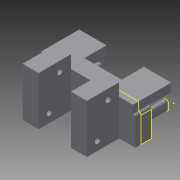
# Autodesk Inventor part: wheelbottomleft
Saved by Autodesk Inventor 2013 SP2 (Build 170200200, 200)
## iProperties
Created: 2015-05-11
Part Number: wheelbottomleft
Document SubType Name: Modeling
Designer: 2016ahoganso
Density: 1 g/cm^3
Material: Generic
Author: 2016ahoganso
Autodesk Inventor part; units mm, degrees
ref_plane "YZ Plane" through (0, 0, 0) normal (1, 0, 0) x (0, 1, 0)
ref_plane "XZ Plane" through (0, 0, 0) normal (0, 1, 0) x (-1, 0, 0)
ref_plane "XY Plane" through (0, 0, 0) normal (0, 0, 1) x (1, 0, 0)
sketch "Sketch1" plane through (0, 0, 0) normal (0, 0, 1) x (1, 0, 0)
  line L0 (2.032, 0) -> (2.032, 0)
  line L1 (4.064, -2.032) -> (4.064, -6.096)
  line L2 (2.032, -8.128) -> (2.032, -8.128)
  line L3 (0, -6.096) -> (0, -2.032)
  arc A0 (2.032, -8.128) -> (4.064, -6.096) centre (2.032, -6.096) ccw
  arc A1 (0, -6.096) -> (2.032, -8.128) centre (2.032, -6.096) ccw
  arc A2 (4.064, -2.032) -> (2.032, 0) centre (2.032, -2.032) ccw
  arc A3 (2.032, 0) -> (0, -2.032) centre (2.032, -2.032) ccw
  line L4 (-8.636, -2.032) -> (-8.636, -6.096)
  line L5 (-12.7, -6.096) -> (-12.7, -2.032)
  arc A4 (-10.668, -8.128) -> (-8.636, -6.096) centre (-10.668, -6.096) ccw
  arc A5 (-12.7, -6.096) -> (-10.668, -8.128) centre (-10.668, -6.096) ccw
  arc A6 (-8.636, -2.032) -> (-10.668, 0) centre (-10.668, -2.032) ccw
  arc A7 (-10.668, 0) -> (-12.7, -2.032) centre (-10.668, -2.032) ccw
  line L6 (8.128, 6.604) -> (-17.018, 6.604)
  line L7 (-17.018, 6.604) -> (-17.018, -15.494)
  line L8 (-17.018, -15.494) -> (8.128, -15.494)
  line L9 (8.128, 6.604) -> (8.128, -15.494)
  line L10 (8.128, -15.494) -> (-17.018, -15.494)
  line L11 (-17.018, -15.494) -> (-17.018, -19.144)
  line L12 (-17.018, -19.144) -> (8.128, -19.144)
  line L13 (8.128, -19.144) -> (8.128, -15.494)
  dimension "d15" = 3.65
  constraints: 28 end point, 16 point on circle, 12 tangent, 8 centre point, 6 parallel, 4 perpendicular, 3 horizontal, 2 equal radius
  measures "d15" distance between parallel lines of L10 L12
surface "Composite1"
surface "Composite2"
surface "Composite3"
surface "Composite4"
surface "Composite5"
surface "Composite6"
surface "Composite7"
surface "Composite8"
surface "Composite9"
surface "Composite10"
extrude "Extrusion2" add sketch "Sketch1" along normal blind 17.526 draft -1 contours L1 A0 A1 L3 A3 A2 | L4 A4 A5 L5 A7 A6
sketch "Sketch2" plane through (0, 0, 17.526) normal (0, 0, 1) x (1, 0, 0)
  line L0 (6.096, 6.858) -> (-15.24, 6.858)
  line L1 (-17.272, 4.826) -> (-17.272, -15.24)
  line L2 (-17.272, -15.24) -> (8.128, -15.24)
  line L3 (8.128, -15.24) -> (8.128, 4.826)
  arc A0 (8.128, 4.826) -> (6.096, 6.858) centre (6.096, 4.826) ccw
  line L4 (0.3059, -6.096) -> (0.3059, -2.032) projected
  line L5 (-17.272, 4.2146) -> (-17.272, 6.858)
  line L6 (-17.272, 6.858) -> (-15.24, 6.858)
  point P0 (0, 0)
  constraints: 12 end point, 3 parallel, 2 point on circle, 2 tangent, 1 centre point, 1 collinear, 1 horizontal, 1 perpendicular, 1 point on line
extrude "Extrusion3" add sketch "Sketch2" along normal blind 6.35
sketch "Sketch3" plane through (0, 0, 23.876) normal (0, 0, 1) x (1, 0, 0)
  line L0 (-15.24, 6.858) -> (6.344, 6.858)
  line L1 (6.344, 6.858) -> (6.344, 13.208)
  line L2 (6.344, 13.208) -> (-15.24, 13.208)
  line L3 (-15.24, 13.208) -> (-15.24, 6.858)
  point P0 (0, 0)
  dimension "d27" = 6.35
  constraints: 8 end point, 2 parallel, 1 horizontal, 1 perpendicular
  measures "d27" distance of L2.end L0.start
extrude "Extrusion4" add sketch "Sketch3" against normal blind 23.876
sketch "Sketch4" plane through (0, 0, 0) normal (0, 0, -1) x (-1, 0, 0)
  arc A0 (-4.064, -6.096) -> (0, -6.096) centre (-2.032, -6.096) ccw projected
  line L0 (0, -6.096) -> (0, -2.032) projected
  arc A1 (0, -2.032) -> (-4.064, -2.032) centre (-2.032, -2.032) ccw projected
  line L1 (-4.064, -2.032) -> (-4.064, -6.096) projected
fillet "Fillet1" radius 1.524 8 edges at (4.064, -4.064, 0) (2.032, -8.128, 0) (0, -4.064, 0) (2.032, 0, 0) (-8.636, -4.064, 0) (-10.668, 0, 0) (-12.7, -4.064, 0) (-10.668, -8.128, 0)
sketch "Sketch5" plane through (0, 0, 23.876) normal (0, 0, 1) x (1, 0, 0)
  arc A0 (-15.24, 6.858) -> (-17.272, 4.826) centre (-15.24, 4.826) ccw projected
  line L0 (-17.272, -15.24) -> (-17.272, 6.858) projected
  line L1 (8.128, -15.24) -> (-17.272, -15.24) projected
  line L2 (8.128, 4.826) -> (8.128, -15.24) projected
  arc A1 (8.128, 4.826) -> (6.096, 6.858) centre (6.096, 4.826) ccw projected
  line L3 (6.096, 6.858) -> (6.344, 6.858) projected
  line L4 (6.344, 6.858) -> (6.344, 13.208) projected
  line L5 (6.344, 13.208) -> (-15.24, 13.208) projected
  line L6 (-15.24, 13.208) -> (-15.24, 6.858) projected
  point P0 (0, 0)
extrude "Extrusion5" add sketch "Sketch5" along normal blind 1.9304
sketch "Sketch7" plane through (0, 0, 25.8064) normal (0, 0, 1) x (1, 0, 0)
  line L0 (-15.24, 6.858) -> (-15.24, 13.208) projected
  arc A0 (-15.24, 6.858) -> (-17.272, 4.826) centre (-15.24, 4.826) ccw projected
  line L1 (-17.272, -15.24) -> (-17.272, 4.826) projected
  line L2 (8.128, -15.24) -> (-17.272, -15.24) projected
  line L3 (8.128, 4.826) -> (8.128, -15.24) projected
  arc A1 (8.128, 4.826) -> (6.096, 6.858) centre (6.096, 4.826) ccw projected
  line L4 (6.344, 6.858) -> (6.096, 6.858) projected
  line L5 (6.344, 13.208) -> (6.344, 6.858) projected
  line L6 (-15.24, 13.208) -> (6.344, 13.208) projected
  line L7 (-4.451, 10.033) -> (-4.451, -12.7593)
  line L8 (-17.272, 4.826) -> (-17.272, 6.858)
  line L9 (-17.272, 6.858) -> (-15.24, 6.858)
  point P0 (0, 0)
  constraints: 6 end point, 2 tangent, 1 parallel, 1 perpendicular
sketch "Sketch8" plane through (8.128, -15.24, 17.526) normal (1, 0, 0) x (0, 0, -1)
  line L0 (0, 0) -> (-8.2804, 0) projected
  line L1 (0, 20.066) -> (0, 0) projected
  line L2 (0, 20.066) -> (-8.2804, 20.066) projected
  line L3 (-8.2804, 20.066) -> (-8.2804, 0) projected
  point P0 (17.526, 15.24)
sketch "Sketch9" plane through (0, 0, 25.8064) normal (0, 0, 1) x (1, 0, 0)
  line L0 (-15.24, 6.858) -> (-15.24, 13.208) projected
  arc A0 (-15.24, 6.858) -> (-17.272, 4.826) centre (-15.24, 4.826) ccw projected
  line L1 (-17.272, -15.24) -> (-17.272, 4.826) projected
  line L2 (8.128, -15.24) -> (-17.272, -15.24) projected
  line L3 (8.128, 4.826) -> (8.128, -15.24) projected
  arc A1 (8.128, 4.826) -> (6.096, 6.858) centre (6.096, 4.826) ccw projected
  line L4 (6.344, 6.858) -> (6.096, 6.858) projected
  line L5 (6.344, 13.208) -> (6.344, 6.858) projected
  line L6 (-15.24, 13.208) -> (6.344, 13.208) projected
  point P0 (0, 0)
extrude "Extrusion6" add sketch "Sketch9" along normal blind 4.4196
sketch "Sketch10" plane through (0, 0, 23.876) normal (0, 0, 1) x (1, 0, 0)
  arc A0 (-15.24, 6.858) -> (-17.272, 4.826) centre (-15.24, 4.826) ccw projected
  line L0 (-17.272, 6.858) -> (-15.24, 6.858) projected
  line L1 (-17.272, 4.826) -> (-17.272, 6.858) projected
  point P0 (0, 0)
extrude "Extrusion7" add sketch "Sketch10" along normal blind 6.35
sketch "Sketch11" plane through (-17.272, 6.858, 17.526) normal (0, 1, 0) x (1, 0, 0)
  line L0 (2.032, -12.7) -> (2.032, 0) projected
  line L1 (0, 0) -> (2.032, 0) projected
  line L2 (0, 0) -> (0, -12.7) projected
  line L3 (0, -12.7) -> (2.032, -12.7) projected
  point P0 (17.272, 17.526)
extrude "Extrusion8" add sketch "Sketch11" along normal blind 6.35
sketch "Sketch12" plane through (0, 0, 30.226) normal (0, 0, 1) x (1, 0, 0)
  line L0 (-17.272, -15.24) -> (-17.272, 13.208) projected
  line L1 (8.128, -15.24) -> (-17.272, -15.24) projected
  line L2 (-17.272, 13.208) -> (-10.922, 13.208)
  line L3 (-10.922, 13.208) -> (-10.922, -15.24)
  line L4 (-10.922, -15.24) -> (-17.272, -15.24)
  line L5 (-17.272, -15.24) -> (-17.272, 13.208)
  point P0 (0, 0)
  dimension "d41" = 6.35
  constraints: 8 end point, 2 parallel, 1 horizontal, 1 perpendicular, 1 point on line
  measures "d41" distance between parallel lines of L0 L3
extrude "Extrusion9" add sketch "Sketch12" along normal blind 25.4
sketch "Sketch13" plane through (0, 0, 30.226) normal (0, 0, 1) x (1, 0, 0)
  line L0 (-10.922, 13.208) -> (-10.922, -15.24) projected
  line L1 (8.128, -15.24) -> (-10.922, -15.24) projected
  line L2 (-10.922, 13.208) -> (-4.572, 13.208)
  line L3 (-4.572, 13.208) -> (-4.572, -15.24)
  line L4 (-4.572, -15.24) -> (-10.922, -15.24)
  line L5 (-10.922, -15.24) -> (-10.922, 13.208)
  point P0 (0, 0)
  dimension "d44" = 6.35
  constraints: 8 end point, 2 parallel, 1 horizontal, 1 perpendicular, 1 point on line
  measures "d44" distance between parallel lines of L3 L0
extrude "Extrusion10" add sketch "Sketch13" along normal blind 25.4
sketch "Sketch16" plane through (-17.272, -15.24, 17.526) normal (-1, 0, 0) x (0, 0, 1)
  line L0 (0, 0) -> (0, 28.448) projected
  line L1 (0, 0) -> (38.1, 0) projected
  line L2 (0, 28.448) -> (12.7, 28.448)
  line L3 (12.7, 28.448) -> (12.7, 0)
  line L4 (12.7, 0) -> (0, 0)
  line L5 (0, 0) -> (0, 28.448)
  point P0 (-17.526, 15.24)
  dimension "d56" = 12.7
  constraints: 8 end point, 2 parallel, 1 horizontal, 1 perpendicular, 1 point on line
  measures "d56" distance between parallel lines of L3 L5
extrude "Extrusion12" add sketch "Sketch16" along normal blind 12.7
mirror "Mirror1" about plane through (-29.972, -1.016, 23.876) normal (-1, 0, 0)
sketch "Sketch17" plane through (-17.272, -15.24, 30.226) normal (0, 0, 1) x (1, 0, 0)
  line L0 (-27.432, 28.448) -> (2.032, 28.448) projected
  circle A0 centre (-12.7, 14.224) radius 8.001
  point P0 (17.272, 15.24)
  dimension "d59" = 16.002
  constraints: 1 centre point
  measures "d59" diameter of A0
extrude "Extrusion13" cut sketch "Sketch17" against normal blind 1.524
sketch "Sketch18" plane through (-29.972, -1.016, 28.702) normal (0, 0, 1) x (1, 0, 0)
  circle A0 centre (0, 0) radius 8.001 projected
  circle A1 centre (0, 0) radius 5.0165
  point P0 (29.972, 1.016)
  dimension "d62" = 10.033
  constraints: 1 centre point, 1 coincident
  measures "d62" diameter of A1
extrude "Extrusion14" cut sketch "Sketch18" against normal blind 25.4 contours A1
sketch "Sketch19" plane through (-15.24, 13.208, 0) normal (0, 1, 0) x (1, 0, 0)
  line L0 (-40.132, -30.226) -> (-40.132, -55.626) projected
  line L1 (-27.432, -55.626) -> (-40.132, -55.626) projected
  line L2 (-27.432, -55.626) -> (-27.432, -30.226) projected
  line L3 (-2.032, -55.626) -> (-2.032, -30.226) projected
  line L4 (-2.032, -55.626) -> (10.668, -55.626) projected
  line L5 (10.668, -30.226) -> (10.668, -55.626) projected
  line L6 (-40.132, -30.226) -> (-27.432, -30.226)
  line L7 (-2.032, -30.226) -> (-27.432, -30.226) projected
  line L8 (-2.032, -30.226) -> (10.668, -30.226)
  point P0 (15.24, 0)
  constraints: 4 end point, 2 collinear
extrude "Extrusion15" add sketch "Sketch19" along normal blind 9.906
sketch "Sketch20" plane through (-4.572, -15.24, 55.626) normal (1, 0, 0) x (0, 0, -1)
  line L0 (25.4, 0) -> (0, 0) projected
  line L1 (0, 0) -> (0, 38.354) projected
  line L2 (12.7, 21.59) -> (12.7, 0)
  circle A0 centre (16.9333, 30.734) radius 2.0955
  line L3 (0, 0) -> (8.4667, 0)
  line L4 (8.4667, 0) -> (8.4667, 6.858)
  circle A1 centre (8.4667, 6.858) radius 2.0955
  point P0 (55.626, 15.24)
  dimension "d70" = 4.191
  dimension "d71" = 21.59
  dimension "d72" = 8.4667
  dimension "d73" = 6.858
  dimension "d74" = 4.191
  constraints: 6 end point, 2 centre point, 1 coincident, 1 midpoint, 1 perpendicular, 1 point on line
  measures "d70" diameter of A0
  measures "d71" distance of L2.start L2.end
  measures "d72" distance of L0.end L3.end
  measures "d73" distance of L3.end L4.end
  measures "d74" diameter of A1
extrude "Extrusion16" cut sketch "Sketch20" against normal blind 50.8
body "Solid2"
body "Srf1"
body "Srf2"
body "Srf3"
body "Srf4"
body "Srf5"
body "Srf6"
body "Srf7"
body "Srf8"
body "Srf9"
body "Srf10"
